Autodesk Inventor part; units mm, degrees
(part 5 of 5)
sketch "スケッチ5" plane through (0, 0, 0) normal (0, 0, -1) x (-1, 0, 0)
  line L0 (10.3363, -41.0107) -> (10.2968, -40.8767) projected
  line L1 (10.4616, -41.3668) -> (10.3363, -41.0107) projected
  line L2 (10.6138, -41.716) -> (10.4616, -41.3668) projected
  line L3 (10.7842, -42.0605) -> (10.6138, -41.716) projected
  line L4 (10.9697, -42.401) -> (10.7842, -42.0605) projected
  line L5 (11.1684, -42.7378) -> (10.9697, -42.401) projected
  line L6 (11.3792, -43.0711) -> (11.1684, -42.7378) projected
  line L7 (11.6012, -43.4011) -> (11.3792, -43.0711) projected
  line L8 (11.8338, -43.7278) -> (11.6012, -43.4011) projected
  line L9 (12.0764, -44.0514) -> (11.8338, -43.7278) projected
  line L10 (12.3286, -44.3718) -> (12.0764, -44.0514) projected
  line L11 (12.59, -44.689) -> (12.3286, -44.3718) projected
  line L12 (12.8605, -45.0031) -> (12.59, -44.689) projected
  line L13 (13.1396, -45.314) -> (12.8605, -45.0031) projected
  line L14 (13.4272, -45.6216) -> (13.1396, -45.314) projected
  line L15 (13.723, -45.926) -> (13.4272, -45.6216) projected
  line L16 (14.0269, -46.2271) -> (13.723, -45.926) projected
  line L17 (14.3387, -46.5249) -> (14.0269, -46.2271) projected
  line L18 (14.6582, -46.8193) -> (14.3387, -46.5249) projected
  line L19 (14.9854, -47.1103) -> (14.6582, -46.8193) projected
  line L20 (15.32, -47.3978) -> (14.9854, -47.1103) projected
  line L21 (15.6651, -47.2849) -> (15.32, -47.3978) projected
  line L22 (16.0093, -47.1694) -> (15.6651, -47.2849) projected
  line L23 (16.3527, -47.0515) -> (16.0093, -47.1694) projected
  line L24 (16.6952, -46.9311) -> (16.3527, -47.0515) projected
  line L25 (17.0368, -46.8081) -> (16.6952, -46.9311) projected
  line L26 (17.3775, -46.6827) -> (17.0368, -46.8081) projected
  line L27 (17.7172, -46.5548) -> (17.3775, -46.6827) projected
  line L28 (18.0561, -46.4245) -> (17.7172, -46.5548) projected
  line L29 (18.394, -46.2916) -> (18.0561, -46.4245) projected
  line L30 (18.7309, -46.1563) -> (18.394, -46.2916) projected
  line L31 (18.8024, -45.721) -> (18.7309, -46.1563) projected
  line L32 (18.866, -45.2878) -> (18.8024, -45.721) projected
  line L33 (18.9216, -44.8569) -> (18.866, -45.2878) projected
  line L34 (18.969, -44.4283) -> (18.9216, -44.8569) projected
  line L35 (19.0083, -44.0023) -> (18.969, -44.4283) projected
  line L36 (19.0392, -43.579) -> (19.0083, -44.0023) projected
  line L37 (19.0617, -43.1585) -> (19.0392, -43.579) projected
  line L38 (19.0757, -42.7409) -> (19.0617, -43.1585) projected
  line L39 (19.081, -42.3265) -> (19.0757, -42.7409) projected
  line L40 (19.0774, -41.9154) -> (19.081, -42.3265) projected
  line L41 (19.0647, -41.5079) -> (19.0774, -41.9154) projected
  line L42 (19.0425, -41.1041) -> (19.0647, -41.5079) projected
  line L43 (19.0107, -40.7043) -> (19.0425, -41.1041) projected
  line L44 (18.9686, -40.3088) -> (19.0107, -40.7043) projected
  line L45 (18.9158, -39.9179) -> (18.9686, -40.3088) projected
  line L46 (18.8516, -39.5322) -> (18.9158, -39.9179) projected
  line L47 (18.7748, -39.1522) -> (18.8516, -39.5322) projected
  line L48 (18.6839, -38.7788) -> (18.7748, -39.1522) projected
  line L49 (18.576, -38.4134) -> (18.6839, -38.7788) projected
  line L50 (18.4431, -38.0601) -> (18.576, -38.4134) projected
  line L51 (18.3313, -37.804) -> (18.4431, -38.0601) projected
  line L52 (18.2337, -37.5507) -> (18.3313, -37.804) projected
  line L53 (18.1486, -37.3012) -> (18.2337, -37.5507) projected
  line L54 (18.0734, -37.0569) -> (18.1486, -37.3012) projected
  line L55 (18.0133, -36.8155) -> (18.0734, -37.0569) projected
  line L56 (17.9685, -36.5772) -> (18.0133, -36.8155) projected
  line L57 (17.9393, -36.342) -> (17.9685, -36.5772) projected
  line L58 (17.9202, -36.1129) -> (17.9393, -36.342) projected
  line L59 (17.9169, -35.8874) -> (17.9202, -36.1129) projected
  line L60 (17.9314, -35.6648) -> (17.9169, -35.8874) projected
  line L61 (17.9574, -35.4486) -> (17.9314, -35.6648) projected
  line L62 (18.0008, -35.2362) -> (17.9574, -35.4486) projected
  line L63 (18.0614, -35.0282) -> (18.0008, -35.2362) projected
  line L64 (18.1365, -34.8267) -> (18.0614, -35.0282) projected
  line L65 (18.2329, -34.6288) -> (18.1365, -34.8267) projected
  line L66 (18.3447, -34.4386) -> (18.2329, -34.6288) projected
  line L67 (18.4826, -34.2517) -> (18.3447, -34.4386) projected
  line L68 (18.6427, -34.0722) -> (18.4826, -34.2517) projected
  line L69 (18.8473, -33.8913) -> (18.6427, -34.0722) projected
  line L70 (19.1345, -33.6962) -> (18.8473, -33.8913) projected
  line L71 (19.1827, -33.6688) -> (19.1345, -33.6962) projected
  line L72 (19.2308, -33.6413) -> (19.1827, -33.6688) projected
  line L73 (19.2789, -33.6138) -> (19.2308, -33.6413) projected
  line L74 (19.327, -33.5862) -> (19.2789, -33.6138) projected
  line L75 (19.375, -33.5585) -> (19.327, -33.5862) projected
  line L76 (19.423, -33.5307) -> (19.375, -33.5585) projected
  line L77 (19.4709, -33.5029) -> (19.423, -33.5307) projected
  line L78 (19.5188, -33.475) -> (19.4709, -33.5029) projected
  line L79 (19.5667, -33.4471) -> (19.5188, -33.475) projected
  line L80 (19.6145, -33.4191) -> (19.5667, -33.4471) projected
  line L81 (19.9271, -33.2679) -> (19.6145, -33.4191) projected
  line L82 (20.186, -33.1812) -> (19.9271, -33.2679) projected
  line L83 (20.4215, -33.1323) -> (20.186, -33.1812) projected
  line L84 (20.6524, -33.1063) -> (20.4215, -33.1323) projected
  line L85 (20.8729, -33.1046) -> (20.6524, -33.1063) projected
  line L86 (21.0926, -33.12) -> (20.8729, -33.1046) projected
  line L87 (21.3046, -33.1558) -> (21.0926, -33.12) projected
  line L88 (21.515, -33.2073) -> (21.3046, -33.1558) projected
  line L89 (21.7207, -33.2758) -> (21.515, -33.2073) projected
  line L90 (21.9209, -33.3615) -> (21.7207, -33.2758) projected
  line L91 (22.121, -33.4602) -> (21.9209, -33.3615) projected
  line L92 (22.3146, -33.5758) -> (22.121, -33.4602) projected
  line L93 (22.5034, -33.7069) -> (22.3146, -33.5758) projected
  line L94 (22.6925, -33.8498) -> (22.5034, -33.7069) projected
  line L95 (22.8765, -34.0078) -> (22.6925, -33.8498) projected
  line L96 (23.0555, -34.1805) -> (22.8765, -34.0078) projected
  line L97 (23.2294, -34.3678) -> (23.0555, -34.1805) projected
  line L98 (23.403, -34.5662) -> (23.2294, -34.3678) projected
  line L99 (23.5736, -34.7774) -> (23.403, -34.5662) projected
  line L100 (23.7394, -35.0022) -> (23.5736, -34.7774) projected
  line L101 (23.979, -35.294) -> (23.7394, -35.0022) projected
  line L102 (24.2415, -35.5701) -> (23.979, -35.294) projected
  line L103 (24.5194, -35.8356) -> (24.2415, -35.5701) projected
  line L104 (24.8101, -36.092) -> (24.5194, -35.8356) projected
  line L105 (25.1121, -36.3405) -> (24.8101, -36.092) projected
  line L106 (25.4241, -36.5817) -> (25.1121, -36.3405) projected
  line L107 (25.7456, -36.8158) -> (25.4241, -36.5817) projected
  line L108 (26.0759, -37.0434) -> (25.7456, -36.8158) projected
  line L109 (26.4145, -37.2644) -> (26.0759, -37.0434) projected
  line L110 (26.7611, -37.4792) -> (26.4145, -37.2644) projected
  line L111 (27.1153, -37.6879) -> (26.7611, -37.4792) projected
  line L112 (27.4768, -37.8905) -> (27.1153, -37.6879) projected
  line L113 (27.8455, -38.0872) -> (27.4768, -37.8905) projected
  line L114 (28.2209, -38.2779) -> (27.8455, -38.0872) projected
  line L115 (28.603, -38.4628) -> (28.2209, -38.2779) projected
  line L116 (28.9916, -38.6418) -> (28.603, -38.4628) projected
  line L117 (29.3864, -38.815) -> (28.9916, -38.6418) projected
  line L118 (29.7874, -38.9823) -> (29.3864, -38.815) projected
  line L119 (30.1943, -39.1439) -> (29.7874, -38.9823) projected
  line L120 (30.6071, -39.2996) -> (30.1943, -39.1439) projected
  line L121 (30.8927, -39.0755) -> (30.6071, -39.2996) projected
  line L122 (31.1767, -38.8493) -> (30.8927, -39.0755) projected
  line L123 (31.459, -38.621) -> (31.1767, -38.8493) projected
  line L124 (31.7397, -38.3907) -> (31.459, -38.621) projected
  line L125 (32.0186, -38.1583) -> (31.7397, -38.3907) projected
  line L126 (32.2959, -37.924) -> (32.0186, -38.1583) projected
  line L127 (32.5715, -37.6876) -> (32.2959, -37.924) projected
  line L128 (32.8453, -37.4492) -> (32.5715, -37.6876) projected
  line L129 (33.1173, -37.2088) -> (32.8453, -37.4492) projected
  line L130 (33.3877, -36.9664) -> (33.1173, -37.2088) projected
  line L131 (33.306, -36.5329) -> (33.3877, -36.9664) projected
  line L132 (33.2176, -36.1041) -> (33.306, -36.5329) projected
  line L133 (33.1224, -35.6801) -> (33.2176, -36.1041) projected
  line L134 (33.0204, -35.2612) -> (33.1224, -35.6801) projected
  line L135 (32.9116, -34.8475) -> (33.0204, -35.2612) projected
  line L136 (32.7959, -34.4391) -> (32.9116, -34.8475) projected
  line L137 (32.6732, -34.0362) -> (32.7959, -34.4391) projected
  line L138 (32.5436, -33.639) -> (32.6732, -34.0362) projected
  line L139 (32.4068, -33.2478) -> (32.5436, -33.639) projected
  line L140 (32.2628, -32.8628) -> (32.4068, -33.2478) projected
  line L141 (32.1115, -32.4841) -> (32.2628, -32.8628) projected
  line L142 (31.9525, -32.1123) -> (32.1115, -32.4841) projected
  line L143 (31.7858, -31.7475) -> (31.9525, -32.1123) projected
  line L144 (31.6111, -31.3902) -> (31.7858, -31.7475) projected
  line L145 (31.4278, -31.041) -> (31.6111, -31.3902) projected
  line L146 (31.2355, -30.7005) -> (31.4278, -31.041) projected
  line L147 (31.0334, -30.3697) -> (31.2355, -30.7005) projected
  line L148 (30.8202, -30.0499) -> (31.0334, -30.3697) projected
  line L149 (30.5939, -29.7434) -> (30.8202, -30.0499) projected
  line L150 (30.3482, -29.4569) -> (30.5939, -29.7434) projected
  line L151 (30.1555, -29.2545) -> (30.3482, -29.4569) projected
  line L152 (29.9772, -29.0498) -> (30.1555, -29.2545) projected
  line L153 (29.8119, -28.8444) -> (29.9772, -29.0498) projected
  line L154 (29.6577, -28.6406) -> (29.8119, -28.8444) projected
  line L155 (29.5186, -28.4343) -> (29.6577, -28.6406) projected
  line L156 (29.395, -28.2257) -> (29.5186, -28.4343) projected
  line L157 (29.2872, -28.0147) -> (29.395, -28.2257) projected
  line L158 (29.1908, -27.806) -> (29.2872, -28.0147) projected
  line L159 (29.1106, -27.5952) -> (29.1908, -27.806) projected
  line L160 (29.0481, -27.381) -> (29.1106, -27.5952) projected
  line L161 (28.9985, -27.169) -> (29.0481, -27.381) projected
  line L162 (28.9667, -26.9545) -> (28.9985, -27.169) projected
  line L163 (28.9525, -26.7384) -> (28.9667, -26.9545) projected
  line L164 (28.9541, -26.5234) -> (28.9525, -26.7384) projected
  line L165 (28.9771, -26.3044) -> (28.9541, -26.5234) projected
  line L166 (29.0171, -26.0875) -> (28.9771, -26.3044) projected
  line L167 (29.0828, -25.8646) -> (29.0171, -26.0875) projected
  line L168 (29.1718, -25.6412) -> (29.0828, -25.8646) projected
  line L169 (29.3021, -25.4012) -> (29.1718, -25.6412) projected
  line L170 (29.5054, -25.1196) -> (29.3021, -25.4012) projected
  line L171 (29.5412, -25.0774) -> (29.5054, -25.1196) projected
  line L172 (29.5771, -25.0351) -> (29.5412, -25.0774) projected
  line L173 (29.6129, -24.9928) -> (29.5771, -25.0351) projected
  line L174 (29.6486, -24.9504) -> (29.6129, -24.9928) projected
  line L175 (29.6842, -24.908) -> (29.6486, -24.9504) projected
  line L176 (29.7198, -24.8655) -> (29.6842, -24.908) projected
  line L177 (29.7553, -24.823) -> (29.7198, -24.8655) projected
  line L178 (29.7908, -24.7804) -> (29.7553, -24.823) projected
  line L179 (29.8262, -24.7378) -> (29.7908, -24.7804) projected
  line L180 (29.8616, -24.6951) -> (29.8262, -24.7378) projected
  line L181 (30.1036, -24.4461) -> (29.8616, -24.6951) projected
  line L182 (30.3173, -24.2761) -> (30.1036, -24.4461) projected
  line L183 (30.5219, -24.1496) -> (30.3173, -24.2761) projected
  line L184 (30.7299, -24.0462) -> (30.5219, -24.1496) projected
  line L185 (30.9366, -23.9692) -> (30.7299, -24.0462) projected
  line L186 (31.1483, -23.9085) -> (30.9366, -23.9692) projected
  line L187 (31.3597, -23.8696) -> (31.1483, -23.9085) projected
  line L188 (31.575, -23.8461) -> (31.3597, -23.8696) projected
  line L189 (31.7918, -23.8401) -> (31.575, -23.8461) projected
  line L190 (32.0092, -23.8521) -> (31.7918, -23.8401) projected
  line L191 (32.231, -23.8765) -> (32.0092, -23.8521) projected
  line L192 (32.4525, -23.9189) -> (32.231, -23.8765) projected
  line L193 (32.6748, -23.9775) -> (32.4525, -23.9189) projected
  line L194 (32.9013, -24.0471) -> (32.6748, -23.9775) projected
  line L195 (33.1282, -24.1326) -> (32.9013, -24.0471) projected
  line L196 (33.3555, -24.2337) -> (33.1282, -24.1326) projected
  line L197 (33.583, -24.3502) -> (33.3555, -24.2337) projected
  line L198 (33.814, -24.4773) -> (33.583, -24.3502) projected
  line L199 (34.0465, -24.6174) -> (33.814, -24.4773) projected
  line L200 (34.2792, -24.772) -> (34.0465, -24.6174) projected
  line L201 (34.6041, -24.9642) -> (34.2792, -24.772) projected
  line L202 (34.9452, -25.1339) -> (34.6041, -24.9642) projected
  line L203 (35.2972, -25.2883) -> (34.9452, -25.1339) projected
  line L204 (35.6581, -25.4299) -> (35.2972, -25.2883) projected
  line L205 (36.0268, -25.5601) -> (35.6581, -25.4299) projected
  line L206 (36.4025, -25.68) -> (36.0268, -25.5601) projected
  line L207 (36.7847, -25.7901) -> (36.4025, -25.68) projected
  line L208 (37.1729, -25.8909) -> (36.7847, -25.7901) projected
  line L209 (37.5667, -25.9828) -> (37.1729, -25.8909) projected
  line L210 (37.9659, -26.0661) -> (37.5667, -25.9828) projected
  line L211 (38.3701, -26.1411) -> (37.9659, -26.0661) projected
  line L212 (38.7791, -26.2078) -> (38.3701, -26.1411) projected
  line L213 (39.1928, -26.2665) -> (38.7791, -26.2078) projected
  line L214 (39.6108, -26.3174) -> (39.1928, -26.2665) projected
  line L215 (40.0331, -26.3604) -> (39.6108, -26.3174) projected
  line L216 (40.4594, -26.3957) -> (40.0331, -26.3604) projected
  line L217 (40.8897, -26.4234) -> (40.4594, -26.3957) projected
  line L218 (41.3237, -26.4435) -> (40.8897, -26.4234) projected
  line L219 (41.7614, -26.4561) -> (41.3237, -26.4435) projected
  line L220 (42.2025, -26.4613) -> (41.7614, -26.4561) projected
  line L221 (42.3943, -26.153) -> (42.2025, -26.4613) projected
  line L222 (42.5838, -25.8433) -> (42.3943, -26.153) projected
  line L223 (42.771, -25.5322) -> (42.5838, -25.8433) projected
  line L224 (42.9559, -25.2198) -> (42.771, -25.5322) projected
  line L225 (43.1386, -24.9061) -> (42.9559, -25.2198) projected
  line L226 (43.319, -24.591) -> (43.1386, -24.9061) projected
  line L227 (43.4971, -24.2746) -> (43.319, -24.591) projected
  line L228 (43.6728, -23.957) -> (43.4971, -24.2746) projected
  line L229 (43.8463, -23.638) -> (43.6728, -23.957) projected
  line L230 (44.0174, -23.3178) -> (43.8463, -23.638) projected
  line L231 (43.7924, -22.9383) -> (44.0174, -23.3178) projected
  line L232 (43.5626, -22.5656) -> (43.7924, -22.9383) projected
  line L233 (43.3282, -22.1998) -> (43.5626, -22.5656) projected
  line L234 (43.0891, -21.841) -> (43.3282, -22.1998) projected
  line L235 (42.8453, -21.4895) -> (43.0891, -21.841) projected
  line L236 (42.5969, -21.1453) -> (42.8453, -21.4895) projected
  line L237 (42.3439, -20.8086) -> (42.5969, -21.1453) projected
  line L238 (42.0862, -20.4798) -> (42.3439, -20.8086) projected
  line L239 (41.8239, -20.1589) -> (42.0862, -20.4798) projected
  line L240 (41.5569, -19.8464) -> (41.8239, -20.1589) projected
  line L241 (41.2851, -19.5423) -> (41.5569, -19.8464) projected
  line L242 (41.0086, -19.2472) -> (41.2851, -19.5423) projected
  line L243 (40.7272, -18.9615) -> (41.0086, -19.2472) projected
  line L244 (40.4408, -18.6855) -> (40.7272, -18.9615) projected
  line L245 (40.1491, -18.4201) -> (40.4408, -18.6855) projected
  line L246 (39.852, -18.1659) -> (40.1491, -18.4201) projected
  line L247 (39.5489, -17.9241) -> (39.852, -18.1659) projected
  line L248 (39.2392, -17.6965) -> (39.5489, -17.9241) projected
  line L249 (38.9217, -17.4859) -> (39.2392, -17.6965) projected
  line L250 (38.5928, -17.3007) -> (38.9217, -17.4859) projected
  line L251 (38.3425, -17.1764) -> (38.5928, -17.3007) projected
  line L252 (38.105, -17.0451) -> (38.3425, -17.1764) projected
  line L253 (37.8794, -16.9086) -> (38.105, -17.0451) projected
  line L254 (37.6648, -16.7698) -> (37.8794, -16.9086) projected
  line L255 (37.4636, -16.6236) -> (37.6648, -16.7698) projected
  line L256 (37.2761, -16.4698) -> (37.4636, -16.6236) projected
  line L257 (37.1025, -16.3084) -> (37.2761, -16.4698) projected
  line L258 (36.9406, -16.1452) -> (37.1025, -16.3084) projected
  line L259 (36.7931, -15.9746) -> (36.9406, -16.1452) projected
  line L260 (36.6611, -15.7947) -> (36.7931, -15.9746) projected
  line L261 (36.5421, -15.6124) -> (36.6611, -15.7947) projected
  line L262 (36.4388, -15.4218) -> (36.5421, -15.6124) projected
  line L263 (36.3516, -15.2235) -> (36.4388, -15.4218) projected
  line L264 (36.2795, -15.0209) -> (36.3516, -15.2235) projected
  line L265 (36.2262, -14.8073) -> (36.2795, -15.0209) projected
  line L266 (36.1896, -14.5898) -> (36.2262, -14.8073) projected
  line L267 (36.1751, -14.3579) -> (36.1896, -14.5898) projected
  line L268 (36.1824, -14.1175) -> (36.1751, -14.3579) projected
  line L269 (36.2227, -13.8474) -> (36.1824, -14.1175) projected
  line L270 (36.3174, -13.5133) -> (36.2227, -13.8474) projected
  line L271 (36.3367, -13.4614) -> (36.3174, -13.5133) projected
  line L272 (36.3559, -13.4094) -> (36.3367, -13.4614) projected
  line L273 (36.375, -13.3574) -> (36.3559, -13.4094) projected
  line L274 (36.3941, -13.3053) -> (36.375, -13.3574) projected
  line L275 (36.4131, -13.2533) -> (36.3941, -13.3053) projected
  line L276 (36.432, -13.2012) -> (36.4131, -13.2533) projected
  line L277 (36.4508, -13.1491) -> (36.432, -13.2012) projected
  line L278 (36.4696, -13.0969) -> (36.4508, -13.1491) projected
  line L279 (36.4883, -13.0448) -> (36.4696, -13.0969) projected
  line L280 (36.5069, -12.9926) -> (36.4883, -13.0448) projected
  line L281 (36.6492, -12.6758) -> (36.5069, -12.9926) projected
  line L282 (36.7919, -12.4429) -> (36.6492, -12.6758) projected
  line L283 (36.9408, -12.2541) -> (36.7919, -12.4429) projected
  line L284 (37.1009, -12.0858) -> (36.9408, -12.2541) projected
  line L285 (37.2688, -11.9427) -> (37.1009, -12.0858) projected
  line L286 (37.447, -11.8133) -> (37.2688, -11.9427) projected
  line L287 (37.6324, -11.7044) -> (37.447, -11.8133) projected
  line L288 (37.8267, -11.6087) -> (37.6324, -11.7044) projected
  line L289 (38.0283, -11.529) -> (37.8267, -11.6087) projected
  line L290 (38.2367, -11.4659) -> (38.0283, -11.529) projected
  line L291 (38.4534, -11.4129) -> (38.2367, -11.4659) projected
  line L292 (38.6761, -11.377) -> (38.4534, -11.4129) projected
  line L293 (38.905, -11.3561) -> (38.6761, -11.377) projected
  line L294 (39.1417, -11.344) -> (38.905, -11.3561) projected
  line L295 (39.3842, -11.3467) -> (39.1417, -11.344) projected
  line L296 (39.6323, -11.364) -> (39.3842, -11.3467) projected
  line L297 (39.886, -11.3956) -> (39.6323, -11.364) projected
  line L298 (40.1465, -11.4361) -> (39.886, -11.3956) projected
  line L299 (40.4129, -11.4882) -> (40.1465, -11.4361) projected
  line L300 (40.6845, -11.5538) -> (40.4129, -11.4882) projected
  line L301 (41.0555, -11.6234) -> (40.6845, -11.5538) projected
  line L302 (41.4341, -11.6662) -> (41.0555, -11.6234) projected
  line L303 (41.8176, -11.6908) -> (41.4341, -11.6662) projected
  line L304 (42.2052, -11.7005) -> (41.8176, -11.6908) projected
  line L305 (42.5962, -11.6968) -> (42.2052, -11.7005) projected
  line L306 (42.9903, -11.6809) -> (42.5962, -11.6968) projected
  line L307 (43.387, -11.6536) -> (42.9903, -11.6809) projected
  line L308 (43.7863, -11.6156) -> (43.387, -11.6536) projected
  line L309 (44.1878, -11.5673) -> (43.7863, -11.6156) projected
  line L310 (44.5914, -11.509) -> (44.1878, -11.5673) projected
  line L311 (44.9969, -11.4412) -> (44.5914, -11.509) projected
  line L312 (45.4041, -11.3641) -> (44.9969, -11.4412) projected
  line L313 (45.8128, -11.2778) -> (45.4041, -11.3641) projected
  line L314 (46.223, -11.1825) -> (45.8128, -11.2778) projected
  line L315 (46.6346, -11.0786) -> (46.223, -11.1825) projected
  line L316 (47.0473, -10.9659) -> (46.6346, -11.0786) projected
  line L317 (47.4611, -10.8448) -> (47.0473, -10.9659) projected
  line L318 (47.8758, -10.7152) -> (47.4611, -10.8448) projected
  line L319 (48.2914, -10.5774) -> (47.8758, -10.7152) projected
  line L320 (48.7077, -10.4313) -> (48.2914, -10.5774) projected
  line L321 (48.7824, -10.0761) -> (48.7077, -10.4313) projected
  line L322 (48.8546, -9.7203) -> (48.7824, -10.0761) projected
  line L323 (48.9241, -9.3639) -> (48.8546, -9.7203) projected
  line L324 (48.9911, -9.0071) -> (48.9241, -9.3639) projected
  line L325 (49.0554, -8.6498) -> (48.9911, -9.0071) projected
  line L326 (49.1172, -8.292) -> (49.0554, -8.6498) projected
  line L327 (49.1763, -7.9338) -> (49.1172, -8.292) projected
  line L328 (49.2328, -7.5752) -> (49.1763, -7.9338) projected
  line L329 (49.2867, -7.2162) -> (49.2328, -7.5752) projected
  line L330 (49.338, -6.8568) -> (49.2867, -7.2162) projected
  line L331 (48.9968, -6.5771) -> (49.338, -6.8568) projected
  line L332 (48.6534, -6.3055) -> (48.9968, -6.5771) projected
  line L333 (48.308, -6.0419) -> (48.6534, -6.3055) projected
  line L334 (47.9606, -5.7865) -> (48.308, -6.0419) projected
  line L335 (47.6113, -5.5395) -> (47.9606, -5.7865) projected
  line L336 (47.2601, -5.3011) -> (47.6113, -5.5395) projected
  line L337 (46.9072, -5.0713) -> (47.2601, -5.3011) projected
  line L338 (46.5526, -4.8504) -> (46.9072, -5.0713) projected
  line L339 (46.1963, -4.6386) -> (46.5526, -4.8504) projected
  line L340 (45.8385, -4.4362) -> (46.1963, -4.6386) projected
  line L341 (45.4792, -4.2434) -> (45.8385, -4.4362) projected
  line L342 (45.1184, -4.0607) -> (45.4792, -4.2434) projected
  line L343 (44.7563, -3.8884) -> (45.1184, -4.0607) projected
  line L344 (44.3927, -3.7271) -> (44.7563, -3.8884) projected
  line L345 (44.0279, -3.5774) -> (44.3927, -3.7271) projected
  line L346 (43.6617, -3.4402) -> (44.0279, -3.5774) projected
  line L347 (43.2942, -3.3167) -> (43.6617, -3.4402) projected
  line L348 (42.9254, -3.2087) -> (43.2942, -3.3167) projected
  line L349 (42.555, -3.1194) -> (42.9254, -3.2087) projected
  line L350 (42.1825, -3.0578) -> (42.555, -3.1194) projected
  line L351 (41.9049, -3.0266) -> (42.1825, -3.0578) projected
  line L352 (41.6367, -2.9845) -> (41.9049, -3.0266) projected
  line L353 (41.3781, -2.9334) -> (41.6367, -2.9845) projected
  line L354 (41.1289, -2.8764) -> (41.3781, -2.9334) projected
  line L355 (40.8898, -2.8078) -> (41.1289, -2.8764) projected
  line L356 (40.661, -2.7274) -> (40.8898, -2.8078) projected
  line L357 (40.4428, -2.6351) -> (40.661, -2.7274) projected
  line L358 (40.2348, -2.5371) -> (40.4428, -2.6351) projected
  line L359 (40.0379, -2.4272) -> (40.2348, -2.5371) projected
  line L360 (39.8523, -2.3033) -> (40.0379, -2.4272) projected
  line L361 (39.6781, -2.1727) -> (39.8523, -2.3033) projected
  line L362 (39.5158, -2.0289) -> (39.6781, -2.1727) projected
  line L363 (39.366, -1.8725) -> (39.5158, -2.0289) projected
  line L364 (39.2291, -1.7067) -> (39.366, -1.8725) projected
  line L365 (39.1059, -1.5242) -> (39.2291, -1.7067) projected
  line L366 (38.997, -1.3323) -> (39.1059, -1.5242) projected
  line L367 (38.9042, -1.1194) -> (38.997, -1.3323) projected
  line L368 (38.8288, -0.891) -> (38.9042, -1.1194) projected
  line L369 (38.7743, -0.6234) -> (38.8288, -0.891) projected
  line L370 (38.749, -0.2771) -> (38.7743, -0.6234) projected
  line L371 (38.7494, -0.2217) -> (38.749, -0.2771) projected
  line L372 (38.7496, -0.1663) -> (38.7494, -0.2217) projected
  line L373 (38.7498, -0.1108) -> (38.7496, -0.1663) projected
  line L374 (38.75, -0.0554) -> (38.7498, -0.1108) projected
  line L375 (38.75, 0) -> (38.75, -0.0554) projected
  line L376 (38.75, 0.0554) -> (38.75, 0) projected
  line L377 (38.7498, 0.1108) -> (38.75, 0.0554) projected
  line L378 (38.7496, 0.1663) -> (38.7498, 0.1108) projected
  line L379 (38.7494, 0.2217) -> (38.7496, 0.1663) projected
  line L380 (38.749, 0.2771) -> (38.7494, 0.2217) projected
  line L381 (38.7743, 0.6234) -> (38.749, 0.2771) projected
  line L382 (38.8288, 0.891) -> (38.7743, 0.6234) projected
  line L383 (38.9042, 1.1194) -> (38.8288, 0.891) projected
  line L384 (38.997, 1.3323) -> (38.9042, 1.1194) projected
  line L385 (39.1059, 1.5242) -> (38.997, 1.3323) projected
  line L386 (39.2291, 1.7067) -> (39.1059, 1.5242) projected
  line L387 (39.366, 1.8725) -> (39.2291, 1.7067) projected
  line L388 (39.5158, 2.0289) -> (39.366, 1.8725) projected
  line L389 (39.6781, 2.1727) -> (39.5158, 2.0289) projected
  line L390 (39.8523, 2.3033) -> (39.6781, 2.1727) projected
  line L391 (40.0379, 2.4272) -> (39.8523, 2.3033) projected
  line L392 (40.2348, 2.5371) -> (40.0379, 2.4272) projected
  line L393 (40.4428, 2.6351) -> (40.2348, 2.5371) projected
  line L394 (40.661, 2.7274) -> (40.4428, 2.6351) projected
  line L395 (40.8898, 2.8078) -> (40.661, 2.7274) projected
  line L396 (41.1289, 2.8764) -> (40.8898, 2.8078) projected
  line L397 (41.3781, 2.9334) -> (41.1289, 2.8764) projected
  line L398 (41.6367, 2.9845) -> (41.3781, 2.9334) projected
  line L399 (41.9049, 3.0266) -> (41.6367, 2.9845) projected
  line L400 (42.1825, 3.0578) -> (41.9049, 3.0266) projected
  line L401 (42.555, 3.1194) -> (42.1825, 3.0578) projected
  line L402 (42.9254, 3.2087) -> (42.555, 3.1194) projected
  line L403 (43.2942, 3.3167) -> (42.9254, 3.2087) projected
  line L404 (43.6617, 3.4402) -> (43.2942, 3.3167) projected
  line L405 (44.0279, 3.5774) -> (43.6617, 3.4402) projected
  line L406 (44.3927, 3.7271) -> (44.0279, 3.5774) projected
  line L407 (44.7563, 3.8884) -> (44.3927, 3.7271) projected
  line L408 (45.1184, 4.0607) -> (44.7563, 3.8884) projected
  line L409 (45.4792, 4.2434) -> (45.1184, 4.0607) projected
  line L410 (45.8385, 4.4362) -> (45.4792, 4.2434) projected
  line L411 (46.1963, 4.6386) -> (45.8385, 4.4362) projected
  line L412 (46.5526, 4.8504) -> (46.1963, 4.6386) projected
  line L413 (46.9072, 5.0713) -> (46.5526, 4.8504) projected
  line L414 (47.2601, 5.3011) -> (46.9072, 5.0713) projected
  line L415 (47.6113, 5.5395) -> (47.2601, 5.3011) projected
  line L416 (47.9606, 5.7865) -> (47.6113, 5.5395) projected
  line L417 (48.308, 6.0419) -> (47.9606, 5.7865) projected
  line L418 (48.6534, 6.3055) -> (48.308, 6.0419) projected
  line L419 (48.9968, 6.5771) -> (48.6534, 6.3055) projected
  line L420 (49.338, 6.8568) -> (48.9968, 6.5771) projected
  line L421 (49.2867, 7.2162) -> (49.338, 6.8568) projected
  line L422 (49.2328, 7.5752) -> (49.2867, 7.2162) projected
  line L423 (49.1763, 7.9338) -> (49.2328, 7.5752) projected
  line L424 (49.1172, 8.292) -> (49.1763, 7.9338) projected
  line L425 (49.0554, 8.6498) -> (49.1172, 8.292) projected
  line L426 (48.9911, 9.0071) -> (49.0554, 8.6498) projected
  line L427 (48.9241, 9.3639) -> (48.9911, 9.0071) projected
  line L428 (48.8546, 9.7203) -> (48.9241, 9.3639) projected
  line L429 (48.7824, 10.0761) -> (48.8546, 9.7203) projected
  line L430 (48.7077, 10.4313) -> (48.7824, 10.0761) projected
  line L431 (48.2914, 10.5774) -> (48.7077, 10.4313) projected
  line L432 (47.8758, 10.7152) -> (48.2914, 10.5774) projected
  line L433 (47.4611, 10.8448) -> (47.8758, 10.7152) projected
  line L434 (47.0473, 10.9659) -> (47.4611, 10.8448) projected
  line L435 (46.6346, 11.0786) -> (47.0473, 10.9659) projected
  line L436 (46.223, 11.1825) -> (46.6346, 11.0786) projected
  line L437 (45.8128, 11.2778) -> (46.223, 11.1825) projected
  line L438 (45.4041, 11.3641) -> (45.8128, 11.2778) projected
  line L439 (44.9969, 11.4412) -> (45.4041, 11.3641) projected
  line L440 (44.5914, 11.509) -> (44.9969, 11.4412) projected
  line L441 (44.1878, 11.5673) -> (44.5914, 11.509) projected
  line L442 (43.7863, 11.6156) -> (44.1878, 11.5673) projected
  line L443 (43.387, 11.6536) -> (43.7863, 11.6156) projected
  line L444 (42.9903, 11.6809) -> (43.387, 11.6536) projected
  line L445 (42.5962, 11.6968) -> (42.9903, 11.6809) projected
  line L446 (42.2052, 11.7005) -> (42.5962, 11.6968) projected
  line L447 (41.8176, 11.6908) -> (42.2052, 11.7005) projected
  line L448 (41.4341, 11.6662) -> (41.8176, 11.6908) projected
  line L449 (41.0555, 11.6234) -> (41.4341, 11.6662) projected
  line L450 (40.6845, 11.5538) -> (41.0555, 11.6234) projected
  line L451 (40.4129, 11.4882) -> (40.6845, 11.5538) projected
  line L452 (40.1465, 11.4361) -> (40.4129, 11.4882) projected
  line L453 (39.886, 11.3956) -> (40.1465, 11.4361) projected
  line L454 (39.6323, 11.364) -> (39.886, 11.3956) projected
  line L455 (39.3842, 11.3467) -> (39.6323, 11.364) projected
  line L456 (39.1417, 11.344) -> (39.3842, 11.3467) projected
  line L457 (38.905, 11.3561) -> (39.1417, 11.344) projected
  line L458 (38.6761, 11.377) -> (38.905, 11.3561) projected
  line L459 (38.4534, 11.4129) -> (38.6761, 11.377) projected
  line L460 (38.2367, 11.4659) -> (38.4534, 11.4129) projected
  line L461 (38.0283, 11.529) -> (38.2367, 11.4659) projected
  line L462 (37.8267, 11.6087) -> (38.0283, 11.529) projected
  line L463 (37.6324, 11.7044) -> (37.8267, 11.6087) projected
  line L464 (37.447, 11.8133) -> (37.6324, 11.7044) projected
  line L465 (37.2688, 11.9427) -> (37.447, 11.8133) projected
  line L466 (37.1009, 12.0858) -> (37.2688, 11.9427) projected
  line L467 (36.9408, 12.2541) -> (37.1009, 12.0858) projected
  line L468 (36.7919, 12.4429) -> (36.9408, 12.2541) projected
  line L469 (36.6492, 12.6758) -> (36.7919, 12.4429) projected
  line L470 (36.5069, 12.9926) -> (36.6492, 12.6758) projected
  line L471 (36.4883, 13.0448) -> (36.5069, 12.9926) projected
  line L472 (36.4696, 13.0969) -> (36.4883, 13.0448) projected
  line L473 (36.4508, 13.1491) -> (36.4696, 13.0969) projected
  line L474 (36.432, 13.2012) -> (36.4508, 13.1491) projected
  line L475 (36.4131, 13.2533) -> (36.432, 13.2012) projected
  line L476 (36.3941, 13.3053) -> (36.4131, 13.2533) projected
  line L477 (36.375, 13.3574) -> (36.3941, 13.3053) projected
  line L478 (36.3559, 13.4094) -> (36.375, 13.3574) projected
  line L479 (36.3367, 13.4614) -> (36.3559, 13.4094) projected
  line L480 (36.3174, 13.5133) -> (36.3367, 13.4614) projected
  line L481 (36.2227, 13.8474) -> (36.3174, 13.5133) projected
  line L482 (36.1824, 14.1175) -> (36.2227, 13.8474) projected
  line L483 (36.1751, 14.3579) -> (36.1824, 14.1175) projected
  line L484 (36.1896, 14.5898) -> (36.1751, 14.3579) projected
  line L485 (36.2262, 14.8073) -> (36.1896, 14.5898) projected
  line L486 (36.2795, 15.0209) -> (36.2262, 14.8073) projected
  line L487 (36.3516, 15.2235) -> (36.2795, 15.0209) projected
  line L488 (36.4388, 15.4218) -> (36.3516, 15.2235) projected
  line L489 (36.5421, 15.6124) -> (36.4388, 15.4218) projected
  line L490 (36.6611, 15.7947) -> (36.5421, 15.6124) projected
  line L491 (36.7931, 15.9746) -> (36.6611, 15.7947) projected
  line L492 (36.9406, 16.1452) -> (36.7931, 15.9746) projected
  line L493 (37.1025, 16.3084) -> (36.9406, 16.1452) projected
  line L494 (37.2761, 16.4698) -> (37.1025, 16.3084) projected
  line L495 (37.4636, 16.6236) -> (37.2761, 16.4698) projected
  line L496 (37.6648, 16.7698) -> (37.4636, 16.6236) projected
  line L497 (37.8794, 16.9086) -> (37.6648, 16.7698) projected
  line L498 (38.105, 17.0451) -> (37.8794, 16.9086) projected
  line L499 (38.3425, 17.1764) -> (38.105, 17.0451) projected
  line L500 (38.5928, 17.3007) -> (38.3425, 17.1764) projected
  line L501 (38.9217, 17.4859) -> (38.5928, 17.3007) projected
  line L502 (39.2392, 17.6965) -> (38.9217, 17.4859) projected
  line L503 (39.5489, 17.9241) -> (39.2392, 17.6965) projected
  line L504 (39.852, 18.1659) -> (39.5489, 17.9241) projected
  line L505 (40.1491, 18.4201) -> (39.852, 18.1659) projected
  line L506 (40.4408, 18.6855) -> (40.1491, 18.4201) projected
  line L507 (40.7272, 18.9615) -> (40.4408, 18.6855) projected
  line L508 (41.0086, 19.2472) -> (40.7272, 18.9615) projected
  line L509 (41.2851, 19.5423) -> (41.0086, 19.2472) projected
  line L510 (41.5569, 19.8464) -> (41.2851, 19.5423) projected
  line L511 (41.8239, 20.1589) -> (41.5569, 19.8464) projected
  line L512 (42.0862, 20.4798) -> (41.8239, 20.1589) projected
  line L513 (42.3439, 20.8086) -> (42.0862, 20.4798) projected
  line L514 (42.5969, 21.1453) -> (42.3439, 20.8086) projected
  line L515 (42.8453, 21.4895) -> (42.5969, 21.1453) projected
  line L516 (43.0891, 21.841) -> (42.8453, 21.4895) projected
  line L517 (43.3282, 22.1998) -> (43.0891, 21.841) projected
  line L518 (43.5626, 22.5656) -> (43.3282, 22.1998) projected
  line L519 (43.7924, 22.9383) -> (43.5626, 22.5656) projected
  line L520 (44.0174, 23.3178) -> (43.7924, 22.9383) projected
  line L521 (43.8463, 23.638) -> (44.0174, 23.3178) projected
  line L522 (43.6728, 23.957) -> (43.8463, 23.638) projected
  line L523 (43.4971, 24.2746) -> (43.6728, 23.957) projected
  line L524 (43.319, 24.591) -> (43.4971, 24.2746) projected
  line L525 (43.1386, 24.9061) -> (43.319, 24.591) projected
  line L526 (42.9559, 25.2198) -> (43.1386, 24.9061) projected
  line L527 (42.771, 25.5322) -> (42.9559, 25.2198) projected
  line L528 (42.5838, 25.8433) -> (42.771, 25.5322) projected
  line L529 (42.3943, 26.153) -> (42.5838, 25.8433) projected
  line L530 (42.2025, 26.4613) -> (42.3943, 26.153) projected
  line L531 (41.7614, 26.4561) -> (42.2025, 26.4613) projected
  line L532 (41.3237, 26.4435) -> (41.7614, 26.4561) projected
  line L533 (40.8897, 26.4234) -> (41.3237, 26.4435) projected
  line L534 (40.4594, 26.3957) -> (40.8897, 26.4234) projected
  line L535 (40.0331, 26.3604) -> (40.4594, 26.3957) projected
  line L536 (39.6108, 26.3174) -> (40.0331, 26.3604) projected
  line L537 (39.1928, 26.2665) -> (39.6108, 26.3174) projected
  line L538 (38.7791, 26.2078) -> (39.1928, 26.2665) projected
  line L539 (38.3701, 26.1411) -> (38.7791, 26.2078) projected
  line L540 (37.9659, 26.0661) -> (38.3701, 26.1411) projected
  line L541 (37.5667, 25.9828) -> (37.9659, 26.0661) projected
  line L542 (37.1729, 25.8909) -> (37.5667, 25.9828) projected
  line L543 (36.7847, 25.7901) -> (37.1729, 25.8909) projected
  line L544 (36.4025, 25.68) -> (36.7847, 25.7901) projected
  line L545 (36.0268, 25.5601) -> (36.4025, 25.68) projected
  line L546 (35.6581, 25.4299) -> (36.0268, 25.5601) projected
  line L547 (35.2972, 25.2883) -> (35.6581, 25.4299) projected
  line L548 (34.9452, 25.1339) -> (35.2972, 25.2883) projected
  line L549 (34.6041, 24.9642) -> (34.9452, 25.1339) projected
  line L550 (34.2792, 24.772) -> (34.6041, 24.9642) projected
  line L551 (34.0465, 24.6174) -> (34.2792, 24.772) projected
  line L552 (33.814, 24.4773) -> (34.0465, 24.6174) projected
  line L553 (33.583, 24.3502) -> (33.814, 24.4773) projected
  line L554 (33.3555, 24.2337) -> (33.583, 24.3502) projected
  line L555 (33.1282, 24.1326) -> (33.3555, 24.2337) projected
  line L556 (32.9013, 24.0471) -> (33.1282, 24.1326) projected
  line L557 (32.6748, 23.9775) -> (32.9013, 24.0471) projected
  line L558 (32.4525, 23.9189) -> (32.6748, 23.9775) projected
  line L559 (32.231, 23.8765) -> (32.4525, 23.9189) projected
  line L560 (32.0092, 23.8521) -> (32.231, 23.8765) projected
  line L561 (31.7918, 23.8401) -> (32.0092, 23.8521) projected
  line L562 (31.575, 23.8461) -> (31.7918, 23.8401) projected
  line L563 (31.3597, 23.8696) -> (31.575, 23.8461) projected
  line L564 (31.1483, 23.9085) -> (31.3597, 23.8696) projected
  line L565 (30.9366, 23.9692) -> (31.1483, 23.9085) projected
  line L566 (30.7299, 24.0462) -> (30.9366, 23.9692) projected
  line L567 (30.5219, 24.1496) -> (30.7299, 24.0462) projected
  line L568 (30.3173, 24.2761) -> (30.5219, 24.1496) projected
  line L569 (30.1036, 24.4461) -> (30.3173, 24.2761) projected
  line L570 (29.8616, 24.6951) -> (30.1036, 24.4461) projected
  line L571 (29.8262, 24.7378) -> (29.8616, 24.6951) projected
  line L572 (29.7908, 24.7804) -> (29.8262, 24.7378) projected
  line L573 (29.7553, 24.823) -> (29.7908, 24.7804) projected
  line L574 (29.7198, 24.8655) -> (29.7553, 24.823) projected
  line L575 (29.6842, 24.908) -> (29.7198, 24.8655) projected
  line L576 (29.6486, 24.9504) -> (29.6842, 24.908) projected
  line L577 (29.6129, 24.9928) -> (29.6486, 24.9504) projected
  line L578 (29.5771, 25.0351) -> (29.6129, 24.9928) projected
  line L579 (29.5412, 25.0774) -> (29.5771, 25.0351) projected
  line L580 (29.5054, 25.1196) -> (29.5412, 25.0774) projected
  line L581 (29.3021, 25.4012) -> (29.5054, 25.1196) projected
  line L582 (29.1718, 25.6412) -> (29.3021, 25.4012) projected
  line L583 (29.0828, 25.8646) -> (29.1718, 25.6412) projected
  line L584 (29.0171, 26.0875) -> (29.0828, 25.8646) projected
  line L585 (28.9771, 26.3044) -> (29.0171, 26.0875) projected
  line L586 (28.9541, 26.5234) -> (28.9771, 26.3044) projected
  line L587 (28.9525, 26.7384) -> (28.9541, 26.5234) projected
  line L588 (28.9667, 26.9545) -> (28.9525, 26.7384) projected
  line L589 (28.9985, 27.169) -> (28.9667, 26.9545) projected
  line L590 (29.0481, 27.381) -> (28.9985, 27.169) projected
  line L591 (29.1106, 27.5952) -> (29.0481, 27.381) projected
  line L592 (29.1908, 27.806) -> (29.1106, 27.5952) projected
  line L593 (29.2872, 28.0147) -> (29.1908, 27.806) projected
  line L594 (29.395, 28.2257) -> (29.2872, 28.0147) projected
  line L595 (29.5186, 28.4343) -> (29.395, 28.2257) projected
  line L596 (29.6577, 28.6406) -> (29.5186, 28.4343) projected
  line L597 (29.8119, 28.8444) -> (29.6577, 28.6406) projected
  line L598 (29.9772, 29.0498) -> (29.8119, 28.8444) projected
  line L599 (30.1555, 29.2545) -> (29.9772, 29.0498) projected
  line L600 (30.3482, 29.4569) -> (30.1555, 29.2545) projected
  line L601 (30.5939, 29.7434) -> (30.3482, 29.4569) projected
  line L602 (30.8202, 30.0499) -> (30.5939, 29.7434) projected
  line L603 (31.0334, 30.3697) -> (30.8202, 30.0499) projected
  line L604 (31.2355, 30.7005) -> (31.0334, 30.3697) projected
  line L605 (31.4278, 31.041) -> (31.2355, 30.7005) projected
  line L606 (31.6111, 31.3902) -> (31.4278, 31.041) projected
  line L607 (31.7858, 31.7475) -> (31.6111, 31.3902) projected
  line L608 (31.9525, 32.1123) -> (31.7858, 31.7475) projected
  line L609 (32.1115, 32.4841) -> (31.9525, 32.1123) projected
  line L610 (32.2628, 32.8628) -> (32.1115, 32.4841) projected
  line L611 (32.4068, 33.2478) -> (32.2628, 32.8628) projected
  line L612 (32.5436, 33.639) -> (32.4068, 33.2478) projected
  line L613 (32.6732, 34.0362) -> (32.5436, 33.639) projected
  line L614 (32.7959, 34.4391) -> (32.6732, 34.0362) projected
  line L615 (32.9116, 34.8475) -> (32.7959, 34.4391) projected
  line L616 (33.0204, 35.2612) -> (32.9116, 34.8475) projected
  line L617 (33.1224, 35.6801) -> (33.0204, 35.2612) projected
  line L618 (33.2176, 36.1041) -> (33.1224, 35.6801) projected
  line L619 (33.306, 36.5329) -> (33.2176, 36.1041) projected
  line L620 (33.3877, 36.9664) -> (33.306, 36.5329) projected
  line L621 (33.1173, 37.2088) -> (33.3877, 36.9664) projected
  line L622 (32.8453, 37.4492) -> (33.1173, 37.2088) projected
  line L623 (32.5715, 37.6876) -> (32.8453, 37.4492) projected
  line L624 (32.2959, 37.924) -> (32.5715, 37.6876) projected
  line L625 (32.0186, 38.1583) -> (32.2959, 37.924) projected
  line L626 (31.7397, 38.3907) -> (32.0186, 38.1583) projected
  line L627 (31.459, 38.621) -> (31.7397, 38.3907) projected
  line L628 (31.1767, 38.8493) -> (31.459, 38.621) projected
  line L629 (30.8927, 39.0755) -> (31.1767, 38.8493) projected
  line L630 (30.6071, 39.2996) -> (30.8927, 39.0755) projected
  line L631 (30.1943, 39.1439) -> (30.6071, 39.2996) projected
  line L632 (29.7874, 38.9823) -> (30.1943, 39.1439) projected
  line L633 (29.3864, 38.815) -> (29.7874, 38.9823) projected
  line L634 (28.9916, 38.6418) -> (29.3864, 38.815) projected
  line L635 (28.603, 38.4628) -> (28.9916, 38.6418) projected
  line L636 (28.2209, 38.2779) -> (28.603, 38.4628) projected
  line L637 (27.8455, 38.0872) -> (28.2209, 38.2779) projected
  line L638 (27.4768, 37.8905) -> (27.8455, 38.0872) projected
  line L639 (27.1153, 37.6879) -> (27.4768, 37.8905) projected
  line L640 (26.7611, 37.4792) -> (27.1153, 37.6879) projected
  line L641 (26.4145, 37.2644) -> (26.7611, 37.4792) projected
  line L642 (26.0759, 37.0434) -> (26.4145, 37.2644) projected
  line L643 (25.7456, 36.8158) -> (26.0759, 37.0434) projected
  line L644 (25.4241, 36.5817) -> (25.7456, 36.8158) projected
  line L645 (25.1121, 36.3405) -> (25.4241, 36.5817) projected
  line L646 (24.8101, 36.092) -> (25.1121, 36.3405) projected
  line L647 (24.5194, 35.8356) -> (24.8101, 36.092) projected
  line L648 (24.2415, 35.5701) -> (24.5194, 35.8356) projected
  line L649 (23.979, 35.294) -> (24.2415, 35.5701) projected
  line L650 (23.7394, 35.0022) -> (23.979, 35.294) projected
  line L651 (-4.3156, 42.2598) -> (-9.1991, 59.2906) projected
  arc A0 (-9.1991, 59.2906) -> (-51.5273, 30.7399) centre (0, 0) ccw projected
  line L652 (-51.5273, 30.7399) -> (-33.9728, 17.0249) projected
  circle A1 centre (-9.3717, 32.6829) radius 1.2295 projected
  circle A2 centre (-26.7924, 20.9325) radius 1.2295 projected
  circle A3 centre (-38.6125, 30.1674) radius 1.2295 projected
  circle A4 centre (-13.5062, 47.1018) radius 1.2295 projected
  line L653 (11.4797, -29.842) -> (0.1321, -14.9781)
  line L654 (-14.6158, 3.3734) -> (-29.7875, 21.369)
  line L655 (-29.7875, 21.369) -> (-59.2243, 44.3676)
  arc A5 (-27.5016, 68.6998) -> (-53.3951, 51.2344) centre (0, 0) ccw
  line L656 (-18.9511, 71.5322) -> (-9.2918, 37.8462)
  line L657 (-2.2045, 34.873) -> (18.4109, 26.1817)
  line L658 (-13.5719, 20.1212) -> (-27.5016, 68.6998)
  line L659 (-53.3951, 51.2344) -> (-13.5719, 20.1212)
  line L660 (-0.018, 0.0211) -> (29.5054, 25.1196) construction
  arc A6 (-1.9627, 2.3054) -> (1.9268, -2.2632) centre (-0.018, 0.0211) ccw
  line L661 (-2.2045, 34.873) -> (3.6161, 14.5742)
  line L662 (-4.3156, 42.2598) -> (-9.1991, 59.2906) projected
  line L663 (22.2957, 22.958) -> (9.228, 11.8327)
  line L664 (0.0518, 4.0205) -> (-1.9627, 2.3054)
  line L665 (1.9268, -2.2632) -> (3.9413, -0.5481)
  line L666 (13.1175, 7.2641) -> (26.1852, 18.3894)
  arc A7 (11.4797, -29.842) -> (26.1852, 18.3894) centre (-0.018, 0.0211) ccw
  arc A8 (22.2957, 22.958) -> (18.4109, 26.1817) centre (-0.018, 0.0211) ccw
  arc A9 (9.228, 11.8327) -> (3.6161, 14.5742) centre (-0.018, 0.0211) ccw
  arc A10 (0.1321, -14.9781) -> (13.1175, 7.2641) centre (-0.018, 0.0211) ccw
  arc A11 (-14.9668, -0.9981) -> (-11.4804, -9.6286) centre (-0.018, 0.0211) ccw
  arc A12 (-14.9878, 0.6496) -> (-14.9859, -0.6499) centre (-0.018, 0.0211) ccw
  arc A13 (-14.8144, 2.3637) -> (-14.9668, 0.9981) centre (-0.018, 0.0211) ccw
  arc A14 (-14.7142, 2.9147) -> (-14.7274, 2.8465) centre (-0.018, 0.0211) ccw
  line L667 (9.2822, -36.8489) -> (10.2968, -40.8767) projected
  line L668 (23.5736, 34.7774) -> (23.7394, 35.0022) projected
  line L669 (23.403, 34.5662) -> (23.5736, 34.7774) projected
  line L670 (23.2294, 34.3678) -> (23.403, 34.5662) projected
  line L671 (23.0555, 34.1805) -> (23.2294, 34.3678) projected
  line L672 (22.8765, 34.0078) -> (23.0555, 34.1805) projected
  line L673 (22.6925, 33.8498) -> (22.8765, 34.0078) projected
  line L674 (22.5034, 33.7069) -> (22.6925, 33.8498) projected
  line L675 (22.3146, 33.5758) -> (22.5034, 33.7069) projected
  line L676 (22.121, 33.4602) -> (22.3146, 33.5758) projected
  line L677 (21.9209, 33.3615) -> (22.121, 33.4602) projected
  line L678 (21.7207, 33.2758) -> (21.9209, 33.3615) projected
  line L679 (21.515, 33.2073) -> (21.7207, 33.2758) projected
  line L680 (21.3046, 33.1558) -> (21.515, 33.2073) projected
  line L681 (21.0926, 33.12) -> (21.3046, 33.1558) projected
  line L682 (20.8729, 33.1046) -> (21.0926, 33.12) projected
  line L683 (20.6524, 33.1063) -> (20.8729, 33.1046) projected
  line L684 (20.4215, 33.1323) -> (20.6524, 33.1063) projected
  line L685 (20.186, 33.1812) -> (20.4215, 33.1323) projected
  line L686 (19.9271, 33.2679) -> (20.186, 33.1812) projected
  line L687 (19.6145, 33.4191) -> (19.9271, 33.2679) projected
  line L688 (19.5667, 33.4471) -> (19.6145, 33.4191) projected
  line L689 (19.5188, 33.475) -> (19.5667, 33.4471) projected
  line L690 (19.4709, 33.5029) -> (19.5188, 33.475) projected
  line L691 (19.423, 33.5307) -> (19.4709, 33.5029) projected
  line L692 (19.375, 33.5585) -> (19.423, 33.5307) projected
  line L693 (19.327, 33.5862) -> (19.375, 33.5585) projected
  line L694 (19.2789, 33.6138) -> (19.327, 33.5862) projected
  line L695 (19.2308, 33.6413) -> (19.2789, 33.6138) projected
  line L696 (19.1827, 33.6688) -> (19.2308, 33.6413) projected
  line L697 (19.1345, 33.6962) -> (19.1827, 33.6688) projected
  line L698 (18.8473, 33.8913) -> (19.1345, 33.6962) projected
  line L699 (18.6427, 34.0722) -> (18.8473, 33.8913) projected
  line L700 (18.4826, 34.2517) -> (18.6427, 34.0722) projected
  line L701 (18.3447, 34.4386) -> (18.4826, 34.2517) projected
  line L702 (18.2329, 34.6288) -> (18.3447, 34.4386) projected
  line L703 (18.1365, 34.8267) -> (18.2329, 34.6288) projected
  line L704 (18.0614, 35.0282) -> (18.1365, 34.8267) projected
  line L705 (18.0008, 35.2362) -> (18.0614, 35.0282) projected
  line L706 (17.9574, 35.4486) -> (18.0008, 35.2362) projected
  line L707 (17.9314, 35.6648) -> (17.9574, 35.4486) projected
  line L708 (17.9169, 35.8874) -> (17.9314, 35.6648) projected
  line L709 (17.9202, 36.1129) -> (17.9169, 35.8874) projected
  line L710 (17.9393, 36.342) -> (17.9202, 36.1129) projected
  line L711 (17.9685, 36.5772) -> (17.9393, 36.342) projected
  line L712 (18.0133, 36.8155) -> (17.9685, 36.5772) projected
  line L713 (18.0734, 37.0569) -> (18.0133, 36.8155) projected
  line L714 (18.1486, 37.3012) -> (18.0734, 37.0569) projected
  line L715 (18.2337, 37.5507) -> (18.1486, 37.3012) projected
  line L716 (18.3313, 37.804) -> (18.2337, 37.5507) projected
  line L717 (18.4431, 38.0601) -> (18.3313, 37.804) projected
  line L718 (18.576, 38.4134) -> (18.4431, 38.0601) projected
  line L719 (18.6839, 38.7788) -> (18.576, 38.4134) projected
  line L720 (18.7748, 39.1522) -> (18.6839, 38.7788) projected
  line L721 (18.8516, 39.5322) -> (18.7748, 39.1522) projected
  line L722 (18.9158, 39.9179) -> (18.8516, 39.5322) projected
  line L723 (18.9686, 40.3088) -> (18.9158, 39.9179) projected
  line L724 (19.0107, 40.7043) -> (18.9686, 40.3088) projected
  line L725 (19.0425, 41.1041) -> (19.0107, 40.7043) projected
  line L726 (19.0647, 41.5079) -> (19.0425, 41.1041) projected
  line L727 (19.0774, 41.9154) -> (19.0647, 41.5079) projected
  line L728 (19.081, 42.3265) -> (19.0774, 41.9154) projected
  line L729 (19.0757, 42.7409) -> (19.081, 42.3265) projected
  line L730 (19.0617, 43.1585) -> (19.0757, 42.7409) projected
  line L731 (19.0392, 43.579) -> (19.0617, 43.1585) projected
  line L732 (19.0083, 44.0023) -> (19.0392, 43.579) projected
  line L733 (18.969, 44.4283) -> (19.0083, 44.0023) projected
  line L734 (18.9216, 44.8569) -> (18.969, 44.4283) projected
  line L735 (18.866, 45.2878) -> (18.9216, 44.8569) projected
  line L736 (18.8024, 45.721) -> (18.866, 45.2878) projected
  line L737 (18.7309, 46.1563) -> (18.8024, 45.721) projected
  line L738 (18.394, 46.2916) -> (18.7309, 46.1563) projected
  line L739 (18.0561, 46.4245) -> (18.394, 46.2916) projected
  line L740 (17.7172, 46.5548) -> (18.0561, 46.4245) projected
  line L741 (17.3775, 46.6827) -> (17.7172, 46.5548) projected
  line L742 (17.0368, 46.8081) -> (17.3775, 46.6827) projected
  line L743 (16.6952, 46.9311) -> (17.0368, 46.8081) projected
  line L744 (16.3527, 47.0515) -> (16.6952, 46.9311) projected
  line L745 (16.0093, 47.1694) -> (16.3527, 47.0515) projected
  line L746 (15.6651, 47.2849) -> (16.0093, 47.1694) projected
  line L747 (15.32, 47.3978) -> (15.6651, 47.2849) projected
  line L748 (15.32, 47.3978) -> (11.6871, 36.1581) projected
  line L749 (11.6871, 36.1581) -> (-4.3156, 42.2598) projected
  line L750 (-33.9728, 17.0249) -> (-11.4682, -9.6686) projected
  line L751 (-11.4682, -9.6686) -> (9.2822, -36.8489) projected
  point P0 (14.7437, 12.5704)
  constraints: 28 end point, 20 point on circle, 10 centre point, 7 parallel, 7 point on line, 4 tangent, 1 coincident, 1 midpoint, 1 perpendicular
extrude "押し出し4" cut sketch "スケッチ5" against normal blind 3 contours L659 A5 L658 A0 | A0 L658 L659 | L653 A10 L666 A7 | L657 A8 L663 A9 L661
fillet "フィレット1" radius 2 18 edges at (13.5719, 20.1212, 1.5) (-9.228, 11.8327, 1.5) (-3.6161, 14.5742, 1.5) (-0.1321, -14.9781, 1.5) (-11.4797, -29.842, 1.5) (-13.1175, 7.2641, 1.5) (-26.1852, 18.3894, 1.5) (-22.2957, 22.958, 1.5) (-18.4109, 26.1817, 1.5) (2.2045, 34.873, 1.5) (9.1991, 59.2906, 1.5) (51.5273, 30.7399, 1.5) (4.3156, 42.2598, 1.5) (-11.6871, 36.1581, 1.5) (-9.2822, -36.8489, 1.5) (33.9728, 17.0249, 1.5) (42.2923, 42.56, 1.5) (23.618, 55.1561, 1.5)
